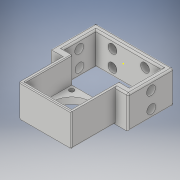
# Autodesk Inventor part: top
Saved by Autodesk Inventor 2018 (Build 220112000, 112)
## iProperties
Created: 2018-09-20
Part Number: top
Material: Generic
Document SubType Name: Modeling
Designer: Iek Man Lei
Density: 1 g/cm^3
Appearance: Default
Author: Iek Man Lei
Autodesk Inventor part; units mm, degrees
ref_plane "YZ Plane" through (0, 0, 0) normal (1, 0, 0) x (0, 1, 0)
ref_plane "XZ Plane" through (0, 0, 0) normal (0, 1, 0) x (-1, 0, 0)
ref_plane "XY Plane" through (0, 0, 0) normal (0, 0, 1) x (1, 0, 0)
sketch "Sketch1" plane through (0, 0, 0) normal (0, 1, 0) x (-1, 0, 0)
  line L0 (30.2857, 41.7143) -> (-17.7143, 41.7143)
  line L1 (-17.7143, 41.7143) -> (-17.7143, -13.2857)
  line L2 (-17.7143, -13.2857) -> (30.2857, -13.2857)
  line L3 (30.2857, -13.2857) -> (30.2857, 41.7143)
  point P0 (0, 0)
  dimension "d0" = 48
  dimension "d1" = 55
  constraints: 8 end point, 2 parallel, 1 horizontal, 1 perpendicular
  measures "d0" distance of L1.end L2.end
  measures "d1" distance of L0.end L1.end
extrude "Extrusion1" add sketch "Sketch1" along normal blind 20
sketch "Sketch5" plane through (0, 20, 0) normal (0, 1, 0) x (1, 0, 0)
  circle A0 centre (-6.2857, -25.4643) radius 11.25
  line L0 (17.7143, 13.2857) -> (-30.2857, 13.2857) projected
  line L1 (-30.2857, 13.2857) -> (-30.2857, -41.7143) projected
  circle A1 centre (5.2143, -36.9643) radius 1.45
  circle A2 centre (-17.7857, -36.9643) radius 1.45
  circle A3 centre (-17.7857, -13.9643) radius 1.45
  circle A4 centre (5.2143, -13.9643) radius 1.45
  line L2 (-30.2857, -41.7143) -> (17.7143, -41.7143) projected
  line L3 (13.8643, -10.7143) -> (-26.4357, -10.7143)
  line L4 (-26.4357, -10.7143) -> (-26.4357, 9.5857)
  line L5 (-26.4357, 9.5857) -> (13.8643, 9.5857)
  line L6 (13.8643, 9.5857) -> (13.8643, -10.7143)
  line L7 (17.7143, -41.7143) -> (17.7143, 13.2857) projected
  line L8 (7.9643, -39.7143) -> (-20.5357, -39.7143)
  line L9 (-20.5357, -39.7143) -> (-20.5357, -11.2143)
  line L10 (-20.5357, -11.2143) -> (7.9643, -11.2143)
  line L11 (7.9643, -11.2143) -> (7.9643, -39.7143)
  point P0 (0, 0)
  point P1 (-13.2857, 11.2857)
  dimension "d14" = 22.5
  dimension "d16" = 24
  dimension "d22" = 2.9
  dimension "d23" = 2.9
  dimension "d24" = 2.9
  dimension "d25" = 2.9
  dimension "d26" = 23
  dimension "d28" = 11.5
  dimension "d29" = 11.5
  dimension "d33" = 40.3
  dimension "d34" = 20.3
  dimension "d36" = 3.85
  dimension "d65" = 14.75
  dimension "d66" = 11.5
  dimension "d67" = 28.5
  dimension "d68" = 28.5
  dimension "d69" = 14.25
  dimension "d83" = 14.25
  dimension "d87" = 3.7
  constraints: 16 end point, 5 centre point, 4 parallel, 2 horizontal, 2 horizontal alignment, 2 perpendicular, 2 vertical alignment, 1 other
  measures "d14" diameter of A0
  measures "d22" diameter of A1
  measures "d23" diameter of A2
  measures "d24" diameter of A3
  measures "d25" diameter of A4
  measures "d26" distance of A4.centre A1.centre
  measures "d28" horizontal distance of A4.centre A0.centre
  measures "d29" horizontal distance of A2.centre A0.centre
  measures "d33" distance of L4.end L5.end
  measures "d34" distance of L3.end L4.end
  measures "d36" distance between parallel lines of L7 L6
  measures "d65" distance from line of L3 A0.centre
  measures "d66" horizontal distance of A0.centre A3.centre
  measures "d67" distance of L9.end L10.end
  measures "d68" distance of L8.end L9.end
  measures "d69" distance from line of A0.centre L9
  measures "d83" distance from line of L8 A0.centre
  measures "d87" distance between parallel lines of L0 L5
extrude "Extrusion5" cut sketch "Sketch5" against normal blind 23 contours A0 | A1 | A2 | A3 | A4 | L3 L4 L5 L6
sketch "Sketch7" plane through (-26.4357, 20, 10.7143) normal (1, 0, 0) x (0, 0, -1)
  circle A0 centre (10, -5) radius 2.75
  line L0 (0, 0) -> (20.3, 0) projected
  line L1 (0, 0) -> (0, -20) projected
  circle A1 centre (10.15, -15) radius 2.75
  line L2 (24, -20) -> (-31, -20) projected
  point P0 (10.7143, -20)
  dimension "d37" = 5.5
  dimension "d38" = 5
  dimension "d39" = 10
  dimension "d79" = 5.5
  dimension "d80" = 5
  constraints: 2 centre point
  measures "d37" diameter of A0
  measures "d38" distance from line of L0 A0.centre
  measures "d39" distance from line of L1 A0.centre
  measures "d79" diameter of A1
  measures "d80" distance from line of L2 A1.centre
extrude "Extrusion6" cut sketch "Sketch7" along normal through all both and the other way through all
sketch "Sketch8" plane through (17.7143, 0, -13.2857) normal (0, 0, -1) x (-1, 0, 0)
  circle A0 centre (34, 15) radius 2.75
  line L0 (10, 19) -> (18, 11)
  circle A1 centre (14, 15) radius 2.75
  line L1 (48, 0) -> (48, 20) projected
  line L2 (0, 0) -> (0, 20) projected
  line L3 (0, 20) -> (48, 20) projected
  line L4 (13.95, 20) -> (13.95, 0) projected
  circle A2 centre (13.95, 5) radius 2.75
  circle A3 centre (34, 5) radius 2.75
  line L5 (0, 0) -> (48, 0) projected
  point P0 (17.7143, 0)
  dimension "d42" = 5.5
  dimension "d43" = 5.5
  dimension "d44" = 20
  dimension "d45" = 14
  dimension "d46" = 14
  dimension "d47" = 5
  dimension "d76" = 5.5
  dimension "d77" = 5.5
  dimension "d78" = 5
  constraints: 4 centre point, 2 end point, 1 horizontal alignment, 1 midpoint, 1 point on line, 1 vertical alignment, 1 other
  measures "d42" diameter of A0
  measures "d43" diameter of A1
  measures "d44" distance of A1.centre A0.centre
  measures "d45" distance from line of L1 A0.centre
  measures "d46" distance from line of L2 A1.centre
  measures "d76" diameter of A2
  measures "d77" diameter of A3
  measures "d78" distance from line of L5 A3.centre
extrude "Extrusion7" cut sketch "Sketch8" against normal blind 7.5 contours A0 | A1 L4 L0 | L0 L4 A1 | L4 A1 L0 | L0 A1 L4 | A2 L4 | L4 A2 | A3
sketch "Sketch9" plane through (0, 0, 0) normal (0, -1, 0) x (1, 0, 0)
  point P0 (0, 0)
sketch "Sketch10" plane through (0, 20, 0) normal (0, 1, 0) x (1, 0, 0)
  line L0 (9.7143, -14.7143) -> (17.7143, -14.7143)
  line L1 (17.7143, -14.7143) -> (17.7143, -41.7143)
  line L2 (17.7143, -41.7143) -> (9.7143, -41.7143)
  line L3 (9.7143, -41.7143) -> (9.7143, -14.7143)
  line L4 (-22.2857, -14.7143) -> (-30.2857, -14.7143)
  line L5 (-30.2857, -14.7143) -> (-30.2857, -41.7143)
  line L6 (-30.2857, -41.7143) -> (-22.2857, -41.7143)
  line L7 (-22.2857, -41.7143) -> (-22.2857, -14.7143)
  point P0 (0, 0)
  dimension "d55" = 8
  dimension "d56" = 8
  dimension "d57" = 27
  constraints: 16 end point, 4 parallel, 2 horizontal, 2 perpendicular, 2 point on line
  measures "d55" distance of L1.end L2.end
  measures "d56" distance of L5.end L6.end
  measures "d57" distance of L0.end L1.end
extrude "Extrusion9" cut sketch "Sketch10" against normal blind 23
sketch "Sketch12" plane through (0, 20, 0) normal (0, 1, 0) x (1, 0, 0)
  point P0 (0, 0)
extrude "Extrusion11" cut sketch "Sketch5" against normal blind 16 contours L8 L9 L10 L11
fillet "Fillet2" radius 0.5 4 edges at (9.7143, 10, 41.7143) (-6.2857, 0, 41.7143) (-22.2857, 10, 41.7143) (-6.2857, 20, 41.7143)
fillet "Fillet3" radius 0.5 4 edges at (7.9643, 20, 25.4643) (-6.2857, 20, 39.7143) (-6.2857, 20, 11.2143) (-20.5357, 20, 25.4643)
fillet "Fillet4" radius 1 23 edges at (-6.2857, 20, -13.2857) (-6.2857, 20, -9.5857) (-26.4357, 20, 0.5643) (-30.2857, 20, 0.7143) (-30.2857, 10, 14.7143) (-30.2857, 10, -13.2857) (-30.2857, 0, 0.7143) (17.7143, 20, 0.7143) (13.8643, 20, 0.5643) (13.7143, 20, 14.7143) (17.7143, 10, -13.2857) (-6.2857, 0, -13.2857) (17.7143, 0, 0.7143) (17.7143, 10, 14.7143) (9.5678, 0.1464, 41.5678) (9.7143, 0, 27.9643) (-22.1393, 0.1464, 41.5678) (-22.2857, 0, 27.9643) (-26.2857, 0, 14.7143) (-6.2857, 0, 10.7143) (-26.4357, 0, 0.5643) (-6.2857, 0, -9.5857) (13.8643, 0, 0.5643)
fillet "Fillet5" radius 0.5 1 edges at (-6.2857, 20, 10.7143)
sketch "Sketch14" plane through (-20.5357, 4, 11.2143) normal (0, 0, 1) x (1, 0, 0)
  line L0 (0, 0) -> (28.5, 0) projected
  line L1 (0, 16) -> (28.5, 16)
  line L2 (28.5, 16) -> (28.5, 0)
  line L3 (28.5, 0) -> (0, 0)
  line L4 (0, 0) -> (0, 16)
  point P0 (20.5357, -4)
  constraints: 8 end point, 2 parallel, 1 horizontal, 1 perpendicular
extrude "Extrusion12" cut sketch "Sketch14" against normal blind 2
fillet "Fillet6" radius 0.5 5 edges at (7.9643, 19.75, 10.7813) (7.9643, 11.75, 10.7143) (-6.2857, 4, 10.7143) (-20.5357, 19.75, 10.7813) (-20.5357, 11.75, 10.7143)
body "Solid1"
